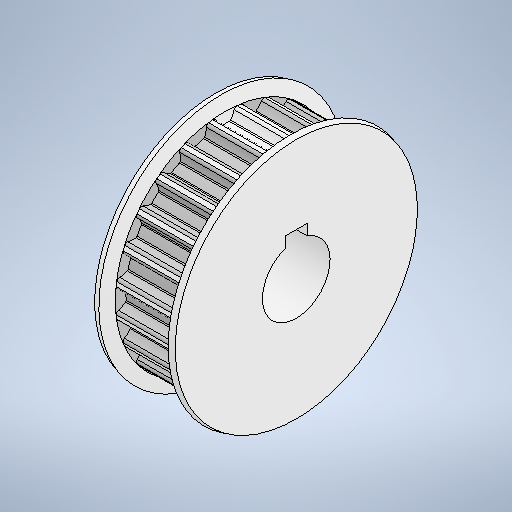
# Autodesk Inventor part: BLPA24S8M150-A-H12_b
Saved by Autodesk Inventor 2025.3 (Build 293356030, 356C)
## iProperties
Category: PARTsolutions
Company: MISUMI
Created: 2025-11-24
Part Number: BLPA24S8M150-A-H12_b
Material: PLA filament
Catalog Web Link: www.3dfindit.com
Description: BLPA__S8M150, BLPA__S8M250, BLPA__S8M300, BLPA__S8M400, BLPK__S8M150, BLPK__S8M250, BLPK__S8M300, BLPK__S8M400, BLPN__S8M150, BLPN__S8M250, BLPN__S8M300, BLPN__S8M400, BLPT__S8M150, BLPT__S8M250, BLPT__S8M300, BLPT__S8M400, BLPM__S8M150, BLPM__S8M250, BLPM__S8M300, BLPM__S8M400, BLPP__S8M150, BLPP__S8M250, BLPP__S8M300, BLPP__S8M400_body-Non-Backlash Timing Pulleys S8M Type
Vendor: MISUMI
Document SubType Name: Modeling
Designer: psAdmin
Manufacturer: MISUMI
Mass: 66.1803 g
Surface Area: 150.756 cm^2
Volume: 55.1502 cm^3
Density: 1.2 g/cm^3
Appearance: 일반
PSOL_IDENT_0: {$CADENAS_DATA/23d-libs/misumi/metric/51_timing_pulleys/blpa_s8m.prj},753 {VTYP=3D},{NB=BLPA24S8M150
PSOL_IDENT_1: -A-H12_b},{LINA=BLPA24S8M150-A-H12},{NN=BLPA__S8M150, BLPA__S8M250, BLPA__S8M300, BLPA__S8M400, BLPK
PSOL_IDENT_2: __S8M150, BLPK__S8M250, BLPK__S8M300, BLPK__S8M400, BLPN__S8M150, BLPN__S8M250, BLPN__S8M300, BLPN__
PSOL_IDENT_3: S8M400, BLPT__S8M150, BLPT__S8M250, BLPT__S8M300, BLPT__S8M400, BLPM__S8M150, BLPM__S8M250, BLPM__S8
PSOL_IDENT_4: M300, BLPM__S8M400, BLPP__S8M150, BLPP__S8M250, BLPP__S8M300, BLPP__S8M400_body},{DATE=08.06.2021 06
PSOL_IDENT_5: :33:40},{GEOMDATE=13.04.2020 01:33:09},{VERSION=},{LINEID=110},{WBVAR=MATP,ST,TNW,PS,SHS,DD,Z,J,Q,R,
PSOL_IDENT_6: S,T,ALT2,M,QSC,QFC,QTC,ALT7,K,KSC,KFC,KTC,ALT11,ZM,ZSC,ZFC,ZTC,ALT1,ALT3,ALT4,ALT5,FC,ALT12,SRG,ALT6
PSOL_IDENT_7: ,TPC,ALT8,BC,ALT9,SLH,ALT10,BTC,TL},{WBNUMERIC=DD,Z,J,Q,R,S,T,QSC,QFC,QTC,K,KSC,KFC,KTC,ZSC,ZFC,ZTC,
PSOL_IDENT_8: FC,SRG,TPC,BC,SLH,BTC,TL}  {NB=BLPA24S8M150-A-H12_b},{LINA=BLPA24S8M150-A-H12},{KT=DUMMY},{PN=BLPA24
PSOL_IDENT_9: S8M150-A-H12},{TYPE=BLPA},{MATP=1},{MATPA=  '1','A7075','2','S45C' },{MATF=A5052},{ST=CA},{STA= 'CA'
PSOL_IDENT_10: , 'Clear Anodize' ,'HAT','Hard Clear Anodize','ENP' , 'Electroless Nickel Plating' },{HARD= - },{NT=
PSOL_IDENT_11: 24},{TNW=S8M150},{BW=15},{A=17},{W=22},{W2=19},{L=37},{L2=34},{PS=A},{PS1='A','B'},{SHS=H},{SHS1='H'
PSOL_IDENT_12: ,'Round Hole','P','Round Hole + Tap','N','New JIS Keywayed Bore + Tap','C','Old JIS Keywayed Bore +
PSOL_IDENT_13: Tap','V','Stepped Hole','Y','Both Ends Stepped Hole','WB','Double Stepped Hole' },{SHS2=-H12},{DD=12
PSOL_IDENT_14: },{DD1=[12:46/1]},{DDH=[12:46/1]},{DDP=[12:40/1]},{DDN=[12:40/1]},{DDC=12,15,16,18,19,20},{DDV=[12:4
PSOL_IDENT_15: 4/1]},{DDF=[12:40/1]},{DDY=[12:44/1]},{DDWB=[12:42/1]},{DD100=12},{DDZ=12},{Z=0},{Z1=0},{ZA=0},{ZB=0
PSOL_IDENT_16: },{ZAB=},{ZQRMIN=14.000},{ZMAX=46},{J=0.0},{J1=0},{JA=0},{JB=0},{JAB=},{Q=0},{WBQMIN=16.000},{Q1=[0]
PSOL_IDENT_17: },{Q2=},{R=0},{WBRMAX=-2.000},{R1=[0]},{R2=},{S=0.0},{S1=[0]},{S2=},{S3=16},{T=0.0},{T1=[0]},{T2=},{
PSOL_IDENT_18: T3=19},{SHMAX=46},{PD=61.12},{OD=59.74},{D=46},{F=67},{E=50},{DE=50},{BJS9=0.000},{TTT=0.0},{NDM=4.0
PSOL_IDENT_19: 00},{WL=22},{ALT2=},{ALT2A='','w/o Side Tapped Hole','-QSC','with QSC (6 Side Tapped Holes)','-QFC','
PSOL_IDENT_20: with QFC (4 Side Tapped Holes)','-QTC','with QTC (3 Side Tapped Holes)'                    },{M=N/A}
PSOL_IDENT_21: ,{MAALG= 'N/A' },{MA= 'N/A' },{MSA= 'N/A' },{MAA=},{QSC=0.0},{QSCA=0},{QSCAA=},{QFC=0.0},{QFCA=0},{Q
PSOL_IDENT_22: FCAA=},{QTC=0.0},{QTCA=0},{QTCAA=},{QC=0.000},{QCMIN=16.000},{QSCMIN=16.000},{QCMAX=46.000},{NDMALT=
PSOL_IDENT_23: 0.000},{QMIN=19.000},{QMAX=43.000},{ALT7=},{ALT7A=    '','w/o Side Through Hole','-KSC','with KSC (6
PSOL_IDENT_24: Side Through Holes)','-KFC','with KFC (4 Side Through Holes)','-KTC','with KTC (3 Side Through Hole
PSOL_IDENT_25: s)'   },{ALT71=    '','w/o Side Through Hole','-KSC','with KSC (6 Side Through Holes)' },{ALT72=    ''
PSOL_IDENT_26: ,'w/o Side Through Hole','-KFC','with KFC (4 Side Through Holes)' },{ALT73=    '','w/o Side Through
PSOL_IDENT_27: Hole','-KTC','with KTC (3 Side Through Holes)' },{K=0.0},{KA=0},{KMAX=13.0},{KSMAX=13.0},{KC=0.000},
PSOL_IDENT_28: {KSC=0.0},{KSCA=0},{KSCAA=},{KFC=0.0},{KFCA=0},{KFCAA=},{KTC=0.0},{KTCA=0},{KTCAA=},{KCMIN=16.000},{
PSOL_IDENT_29: KSCMIN=16.000},{KCMAX=46.000},{KPN=},{ALT11=},{ALT11ALG= '','w/o Side Counterbored','ZSC','with ZSC
PSOL_IDENT_30: (6 Places Side Counterbored)','ZFC','with ZFC (4 Places Side Counterbored)','ZTC','with ZTC (3 Place
PSOL_IDENT_31: s Side Counterbored)' },{ALT11MIN=22.500},{ALT11MAX=39.500},{ZM=N/A},{ZMALG= 'N/A' },{ZMFTALG= 'N/A'
PSOL_IDENT_32: },{ZMSALG= 'N/A' },{ZMDD1=0.0},{ZMDD2=0.0},{ZMHH=0.0},{ZC=0.000},{ZSC=0.0},{ZSCALG=[0]},{ZFC=0.0},{
PSOL_IDENT_33: ZFCALG=[0]},{ZTC=0.0},{ZTCALG=[0]},{ZPCDMIN=0.000},{ZPCDMINALG=0.000},{ZPCDMAX=46.000},{ALT11PN=},{A
PSOL_IDENT_34: LT1=},{ALT1A= '','Not applicable' },{ALT3=},{ALT4=},{ALT4A= '', 'w/o Flange Attached on One Side Onl
PSOL_IDENT_35: y', '-RFC'  , 'with RFC (Flange Attached on The Boss Side Only)', '-LFC'  , 'with LFC (Flange Attach
PSOL_IDENT_36: ed on The Opposite Side Only)' },{ALT5=},{ALT5A='','w/o FC (Flange Cut)','-FC','with FC (Flange Cut)'
PSOL_IDENT_37: },{FCMIN=61.0},{FCMAX=65.0},{FCA=0},{FC=0.0},{FCAA=},{ALT12=},{ALT12ALG= '','Not applicable' },{ALT1
PSOL_IDENT_38: 2ALGALG=46.000},{ALT12DD2=0.000},{ALT12MM=0.000},{ALT12NN=0.000},{SRG=0.0},{SRGALG=[0]},{SRGMAX=0.0}
PSOL_IDENT_39: ,{SRGMAX1=0.000},{DD2=0.0},{MM=0.00},{NN=0.00},{ALT12PN=},{ALT6=},{ALT6A= '','Not applicable' },{TPC=
PSOL_IDENT_40: 0},{TPCA=           0,'N/A'         },{TPCAA=},{ALFA=5.300},{ZUB=5.200},{TT=0.5},{TAP=0.000},{DDD=50
PSOL_IDENT_41: .000},{ALT8=},{ALT8A= '','Not applicable' },{BC=0.0},{BCCA=0},{BCCAMIN=3},{BCCAMAX=14.5},{BCPLANE=11
PSOL_IDENT_42: },{BCAA=},{KTT=23.87},{KYY=6},{PLANE=22},{TIF=1},{LS=3},{WS=4},{ANG=120},{ALT9=},{ALT9A= '','Not app
PSOL_IDENT_43: licable' },{SLH=0},{SLH1=0},{ALT9PN=},{WLBC=22},{KDML=0.0},{ALT10=},{ALT10ALG= '','w/o BTC (Taper fo
PSOL_IDENT_44: r Bearing Holder)','BTC','with BTC (Taper for Bearing Holder)' },{BTC10=14},{TL10=1},{BTC=0},{BTCALG=
PSOL_IDENT_45: 0},{TL=0.0},{TLALG=0},{TLMIN=1.000},{TLMAX=10.000},{ALT10PN=},{WLBCTL=22.000},{AC=-}
NB: BLPA24S8M150-A-H12_b
NN: 0
NT: 24
NBSYN: $PN._b
LINA: BLPA24S8M150-A-H12
CATALOG: Misumi
PN: BLPA24S8M150-A-H12
MATP: A7075
MATF: A5052
ST: Clear Anodize
HARD: -
TNW: S8M150
BW: 15
A: 17
W: 22
L: 37
PS: A
SHS: Round Hole
DD: 12
Z: 0
J: 0
Q: 0
R: 0
S: 0
T: 0
PD: 61.12
OD: 59.74
D: 46
F: 67
E: 50
ALT2: w/o Side Tapped Hole
M: N/A
QSC: 0
QFC: 0
QTC: 0
ALT7: w/o Side Through Hole
K: 0
KSC: 0
KFC: 0
KTC: 0
ALT11: w/o Side Counterbored
ZM: N/A
ZMDD1: 0
ZMDD2: 0
ZMHH: 0
ZSC: 0
ZFC: 0
ZTC: 0
ALT1: Not applicable
ALT3: Flange Attached
ALT4: w/o Flange Attached on One Side Only
ALT5: w/o FC (Flange Cut)
FC: 0
ALT12: Not applicable
SRG: 0
DD2: 0
MM: 0
ALT6: Not applicable
TPC: N/A
ALT8: Not applicable
BC: 0
ALT9: Not applicable
SLH: 0
ALT10: w/o BTC (Taper for Bearing Holder)
BTC: 0
TL: 0
AC: -
SUPPLIER: MISUMI
ARTICLENO: BLPA24S8M150-A-H12_b
BOMINFO: BLPA24S8M150-A-H12
CREATOR: CADENAS GmbH
Title: BLPA24S8M150-A-H12
Author: Cadenas PARTsolutions
Comments: Non-Backlash Timing Pulleys S8M Type
Autodesk Inventor part; units mm, degrees
ref_plane "YZ Plane" through (0, 0, 0) normal (1, 0, 0) x (0, 1, 0)
ref_plane "XZ Plane" through (0, 0, 0) normal (0, 1, 0) x (-1, 0, 0)
ref_plane "XY Plane" through (0, 0, 0) normal (0, 0, 1) x (1, 0, 0)
sketch "Sketch_1" plane through (0, 0, 0) normal (0, 0, 1) x (1, 0, 0)
  line L0 (22, 0) -> (0, 0)
  line L1 (0, 0) -> (0, 33.0859)
  line L2 (0, 33.0859) -> (1.5455, 33.5)
  line L3 (1.5455, 33.5) -> (2.5181, 29.87)
  line L4 (2.5181, 29.87) -> (19.5181, 29.87)
  line L5 (19.5181, 29.87) -> (20.4908, 33.5)
  line L6 (20.4908, 33.5) -> (22.0194, 33.0904)
  line L7 (22.0194, 33.0904) -> (22.0194, 0)
  line L8 (22.0194, 0) -> (0, 0)
  constraints: 18 end point
revolve "Revolution1" add sketch "Sketch_1" angle 360 about axis through (22, 0, 0) along (1, 0, 0)
sketch "Sketch2" plane through (22.0194, 0, 0) normal (1, 0, 0) x (0, 0, -1)
  point P0 (0, 0)
hole "Hole1" at (22.0194, 0, 0) direction (-1, 0, 0) diameter 18.5 depth 13.752
sketch "Sketch_2" plane through (2.5, 0, 0) normal (1, 0, 0) x (0, 0, -1)
  line L0 (-3.3419, 39.8267) -> (-3.3419, 29.6825)
  arc A0 (-2.5318, 29.1246) -> (-3.3419, 29.6825) centre (-3.258, 28.9372) ccw
  arc A1 (-2.5318, 29.1246) -> (-1.5589, 27.1638) centre (2.6, 30.4492) ccw
  arc A2 (-1.5589, 27.1638) -> (-1.2268, 27.0122) centre (-1.245, 27.4117) ccw
  arc A3 (1.2268, 27.0122) -> (-1.2268, 27.0122) centre (0, 0) ccw
  arc A4 (1.2268, 27.0122) -> (1.5589, 27.1638) centre (1.245, 27.4117) ccw
  arc A5 (1.5589, 27.1638) -> (2.5318, 29.1246) centre (-2.6, 30.4492) ccw
  arc A6 (3.3419, 29.6825) -> (2.5318, 29.1246) centre (3.258, 28.9372) ccw
  line L1 (3.3419, 29.6825) -> (3.3419, 39.8267)
  line L2 (3.3419, 39.8267) -> (-3.3419, 39.8267)
  constraints: 14 point on circle, 7 centre point, 6 end point
extrude "Extrusion1" cut sketch "Sketch_2" along normal blind 17
pattern_circular "Circular Pattern1" count 24 over 360 about axis through (2.5, 0, 0) along (1, 0, 0) of "Extrusion1"
sketch "스케치4" plane through (22.0194, 0, 0) normal (1, 0, 0) x (0, 0, -1)
  line L0 (-3, 11.75) -> (3, 11.75)
  line L1 (3, 11.75) -> (3, 6.75)
  line L2 (3, 6.75) -> (-3, 6.75)
  line L3 (-3, 6.75) -> (-3, 11.75)
  line L4 (-3, 11.75) -> (3, 6.75) construction
  line L5 (3, 11.75) -> (-3, 6.75) construction
  circle A0 centre (0, 0) radius 9.25 projected
  point P0 (0, 9.25)
  dimension "d13" = 5
  dimension "d14" = 6
  constraints: 12 end point, 2 midpoint, 2 parallel, 2 vertical alignment, 1 horizontal, 1 perpendicular, 1 other
  measures "d13" distance of L0.end L1.end
  measures "d14" distance of L0.start L0.end
extrude "돌출2" cut sketch "스케치4" against normal up to surface (13.752 mm away) contours L0 L1 A0 L3 | A0 L1 L2 L3 picked at (0.3388, 7.5647)
sketch "스케치5" plane through (0, 0, 0) normal (-1, 0, 0) x (0, 0, 1)
  circle A0 centre (0, 0) radius 33.0859 projected
  constraints: 1 coincident
hole "구멍2" at (0, 0, 0) direction (1, 0, 0) diameter 6.6 end through all clearance for "Socket Head Cap Screw ISO 4762" size "M6" standard "ISO"
body "Solid1"
